Autodesk Inventor part; units mm, degrees
(part 7 of 13)
  line L2860 (13.767, 1.3537) -> (13.3324, 0.9191) construction
  line L2861 (13.3324, 0.9191) -> (13.3324, 0.3832) construction
  spline S914 degree 3 poles (13.3324, 0.3832) (13.3324, -0.1529) (13.767, -0.5874) (14.303, -0.5874) knots 0 0 0 0 1 1 1 1
  line L2862 (13.3324, 0.3832) -> (13.3324, -0.1529) construction
  line L2863 (13.3324, -0.1529) -> (13.767, -0.5874) construction
  line L2864 (13.767, -0.5874) -> (14.303, -0.5874) construction
  spline S915 degree 3 poles (14.303, -0.5874) (14.839, -0.5874) (15.2735, -0.1529) (15.2735, 0.3832) knots 0 0 0 0 1 1 1 1
  line L2865 (14.303, -0.5874) -> (14.839, -0.5874) construction
  line L2866 (14.839, -0.5874) -> (15.2735, -0.1529) construction
  line L2867 (15.2735, -0.1529) -> (15.2735, 0.3832) construction
  spline S916 degree 3 poles (17.8276, 0.3832) (17.8276, 0.9191) (17.3931, 1.3537) (16.8571, 1.3537) knots 0 0 0 0 1 1 1 1
  line L2868 (17.8276, 0.3832) -> (17.8276, 0.9191) construction
  line L2869 (17.8276, 0.9191) -> (17.3931, 1.3537) construction
  line L2870 (17.3931, 1.3537) -> (16.8571, 1.3537) construction
  spline S917 degree 3 poles (16.8571, 1.3537) (16.3211, 1.3537) (15.8866, 0.9191) (15.8866, 0.3832) knots 0 0 0 0 1 1 1 1
  line L2871 (16.8571, 1.3537) -> (16.3211, 1.3537) construction
  line L2872 (16.3211, 1.3537) -> (15.8866, 0.9191) construction
  line L2873 (15.8866, 0.9191) -> (15.8866, 0.3832) construction
  spline S918 degree 3 poles (15.8866, 0.3832) (15.8866, -0.1529) (16.3211, -0.5874) (16.8571, -0.5874) knots 0 0 0 0 1 1 1 1
  line L2874 (15.8866, 0.3832) -> (15.8866, -0.1529) construction
  line L2875 (15.8866, -0.1529) -> (16.3211, -0.5874) construction
  line L2876 (16.3211, -0.5874) -> (16.8571, -0.5874) construction
  spline S919 degree 3 poles (16.8571, -0.5874) (17.3931, -0.5874) (17.8276, -0.1529) (17.8276, 0.3832) knots 0 0 0 0 1 1 1 1
  line L2877 (16.8571, -0.5874) -> (17.3931, -0.5874) construction
  line L2878 (17.3931, -0.5874) -> (17.8276, -0.1529) construction
  line L2879 (17.8276, -0.1529) -> (17.8276, 0.3832) construction
  spline S920 degree 3 poles (17.8276, 2.9373) (17.8276, 3.4732) (17.3931, 3.9078) (16.8571, 3.9078) knots 0 0 0 0 1 1 1 1
  line L2880 (17.8276, 2.9373) -> (17.8276, 3.4732) construction
  line L2881 (17.8276, 3.4732) -> (17.3931, 3.9078) construction
  line L2882 (17.3931, 3.9078) -> (16.8571, 3.9078) construction
  spline S921 degree 3 poles (16.8571, 3.9078) (16.3211, 3.9078) (15.8866, 3.4732) (15.8866, 2.9373) knots 0 0 0 0 1 1 1 1
  line L2883 (16.8571, 3.9078) -> (16.3211, 3.9078) construction
  line L2884 (16.3211, 3.9078) -> (15.8866, 3.4732) construction
  line L2885 (15.8866, 3.4732) -> (15.8866, 2.9373) construction
  spline S922 degree 3 poles (15.8866, 2.9373) (15.8866, 2.4013) (16.3211, 1.9667) (16.8571, 1.9667) knots 0 0 0 0 1 1 1 1
  line L2886 (15.8866, 2.9373) -> (15.8866, 2.4013) construction
  line L2887 (15.8866, 2.4013) -> (16.3211, 1.9667) construction
  line L2888 (16.3211, 1.9667) -> (16.8571, 1.9667) construction
  spline S923 degree 3 poles (16.8571, 1.9667) (17.3931, 1.9667) (17.8276, 2.4013) (17.8276, 2.9373) knots 0 0 0 0 1 1 1 1
  line L2889 (16.8571, 1.9667) -> (17.3931, 1.9667) construction
  line L2890 (17.3931, 1.9667) -> (17.8276, 2.4013) construction
  line L2891 (17.8276, 2.4013) -> (17.8276, 2.9373) construction
  spline S924 degree 3 poles (20.3818, 2.9373) (20.3818, 3.4732) (19.9472, 3.9078) (19.4112, 3.9078) knots 0 0 0 0 1 1 1 1
  line L2892 (20.3818, 2.9373) -> (20.3818, 3.4732) construction
  line L2893 (20.3818, 3.4732) -> (19.9472, 3.9078) construction
  line L2894 (19.9472, 3.9078) -> (19.4112, 3.9078) construction
  spline S925 degree 3 poles (19.4112, 3.9078) (18.8752, 3.9078) (18.4407, 3.4732) (18.4407, 2.9373) knots 0 0 0 0 1 1 1 1
  line L2895 (19.4112, 3.9078) -> (18.8752, 3.9078) construction
  line L2896 (18.8752, 3.9078) -> (18.4407, 3.4732) construction
  line L2897 (18.4407, 3.4732) -> (18.4407, 2.9373) construction
  spline S926 degree 3 poles (18.4407, 2.9373) (18.4407, 2.4013) (18.8752, 1.9667) (19.4112, 1.9667) knots 0 0 0 0 1 1 1 1
  line L2898 (18.4407, 2.9373) -> (18.4407, 2.4013) construction
  line L2899 (18.4407, 2.4013) -> (18.8752, 1.9667) construction
  line L2900 (18.8752, 1.9667) -> (19.4112, 1.9667) construction
  spline S927 degree 3 poles (19.4112, 1.9667) (19.9472, 1.9667) (20.3818, 2.4013) (20.3818, 2.9373) knots 0 0 0 0 1 1 1 1
  line L2901 (19.4112, 1.9667) -> (19.9472, 1.9667) construction
  line L2902 (19.9472, 1.9667) -> (20.3818, 2.4013) construction
  line L2903 (20.3818, 2.4013) -> (20.3818, 2.9373) construction
  spline S928 degree 3 poles (26.767, 0.3832) (26.767, 0.9191) (26.3325, 1.3537) (25.7965, 1.3537) knots 0 0 0 0 1 1 1 1
  line L2904 (26.767, 0.3832) -> (26.767, 0.9191) construction
  line L2905 (26.767, 0.9191) -> (26.3325, 1.3537) construction
  line L2906 (26.3325, 1.3537) -> (25.7965, 1.3537) construction
  spline S929 degree 3 poles (25.7965, 1.3537) (25.2605, 1.3537) (24.8259, 0.9191) (24.8259, 0.3832) knots 0 0 0 0 1 1 1 1
  line L2907 (25.7965, 1.3537) -> (25.2605, 1.3537) construction
  line L2908 (25.2605, 1.3537) -> (24.8259, 0.9191) construction
  line L2909 (24.8259, 0.9191) -> (24.8259, 0.3832) construction
  spline S930 degree 3 poles (24.8259, 0.3832) (24.8259, -0.1529) (25.2605, -0.5874) (25.7965, -0.5874) knots 0 0 0 0 1 1 1 1
  line L2910 (24.8259, 0.3832) -> (24.8259, -0.1529) construction
  line L2911 (24.8259, -0.1529) -> (25.2605, -0.5874) construction
  line L2912 (25.2605, -0.5874) -> (25.7965, -0.5874) construction
  spline S931 degree 3 poles (25.7965, -0.5874) (26.3325, -0.5874) (26.767, -0.1529) (26.767, 0.3832) knots 0 0 0 0 1 1 1 1
  line L2913 (25.7965, -0.5874) -> (26.3325, -0.5874) construction
  line L2914 (26.3325, -0.5874) -> (26.767, -0.1529) construction
  line L2915 (26.767, -0.1529) -> (26.767, 0.3832) construction
  spline S932 degree 3 poles (24.2129, 0.3832) (24.2129, 0.9191) (23.7784, 1.3537) (23.2424, 1.3537) knots 0 0 0 0 1 1 1 1
  line L2916 (24.2129, 0.3832) -> (24.2129, 0.9191) construction
  line L2917 (24.2129, 0.9191) -> (23.7784, 1.3537) construction
  line L2918 (23.7784, 1.3537) -> (23.2424, 1.3537) construction
  spline S933 degree 3 poles (23.2424, 1.3537) (22.7064, 1.3537) (22.2718, 0.9191) (22.2718, 0.3832) knots 0 0 0 0 1 1 1 1
  line L2919 (23.2424, 1.3537) -> (22.7064, 1.3537) construction
  line L2920 (22.7064, 1.3537) -> (22.2718, 0.9191) construction
  line L2921 (22.2718, 0.9191) -> (22.2718, 0.3832) construction
  spline S934 degree 3 poles (22.2718, 0.3832) (22.2718, -0.1529) (22.7064, -0.5874) (23.2424, -0.5874) knots 0 0 0 0 1 1 1 1
  line L2922 (22.2718, 0.3832) -> (22.2718, -0.1529) construction
  line L2923 (22.2718, -0.1529) -> (22.7064, -0.5874) construction
  line L2924 (22.7064, -0.5874) -> (23.2424, -0.5874) construction
  spline S935 degree 3 poles (23.2424, -0.5874) (23.7784, -0.5874) (24.2129, -0.1529) (24.2129, 0.3832) knots 0 0 0 0 1 1 1 1
  line L2925 (23.2424, -0.5874) -> (23.7784, -0.5874) construction
  line L2926 (23.7784, -0.5874) -> (24.2129, -0.1529) construction
  line L2927 (24.2129, -0.1529) -> (24.2129, 0.3832) construction
  spline S936 degree 3 poles (21.6588, 0.3832) (21.6588, 0.9191) (21.2243, 1.3537) (20.6882, 1.3537) knots 0 0 0 0 1 1 1 1
  line L2928 (21.6588, 0.3832) -> (21.6588, 0.9191) construction
  line L2929 (21.6588, 0.9191) -> (21.2243, 1.3537) construction
  line L2930 (21.2243, 1.3537) -> (20.6882, 1.3537) construction
  spline S937 degree 3 poles (20.6882, 1.3537) (20.1523, 1.3537) (19.7177, 0.9191) (19.7177, 0.3832) knots 0 0 0 0 1 1 1 1
  line L2931 (20.6882, 1.3537) -> (20.1523, 1.3537) construction
  line L2932 (20.1523, 1.3537) -> (19.7177, 0.9191) construction
  line L2933 (19.7177, 0.9191) -> (19.7177, 0.3832) construction
  spline S938 degree 3 poles (19.7177, 0.3832) (19.7177, -0.1529) (20.1523, -0.5874) (20.6882, -0.5874) knots 0 0 0 0 1 1 1 1
  line L2934 (19.7177, 0.3832) -> (19.7177, -0.1529) construction
  line L2935 (19.7177, -0.1529) -> (20.1523, -0.5874) construction
  line L2936 (20.1523, -0.5874) -> (20.6882, -0.5874) construction
  spline S939 degree 3 poles (20.6882, -0.5874) (21.2243, -0.5874) (21.6588, -0.1529) (21.6588, 0.3832) knots 0 0 0 0 1 1 1 1
  line L2937 (20.6882, -0.5874) -> (21.2243, -0.5874) construction
  line L2938 (21.2243, -0.5874) -> (21.6588, -0.1529) construction
  line L2939 (21.6588, -0.1529) -> (21.6588, 0.3832) construction
  spline S940 degree 3 poles (20.3818, 5.4914) (20.3818, 6.0273) (19.9472, 6.4619) (19.4112, 6.4619) knots 0 0 0 0 1 1 1 1
  line L2940 (20.3818, 5.4914) -> (20.3818, 6.0273) construction
  line L2941 (20.3818, 6.0273) -> (19.9472, 6.4619) construction
  line L2942 (19.9472, 6.4619) -> (19.4112, 6.4619) construction
  spline S941 degree 3 poles (19.4112, 6.4619) (18.8752, 6.4619) (18.4407, 6.0273) (18.4407, 5.4914) knots 0 0 0 0 1 1 1 1
  line L2943 (19.4112, 6.4619) -> (18.8752, 6.4619) construction
  line L2944 (18.8752, 6.4619) -> (18.4407, 6.0273) construction
  line L2945 (18.4407, 6.0273) -> (18.4407, 5.4914) construction
  spline S942 degree 3 poles (18.4407, 5.4914) (18.4407, 4.9554) (18.8752, 4.5208) (19.4112, 4.5208) knots 0 0 0 0 1 1 1 1
  line L2946 (18.4407, 5.4914) -> (18.4407, 4.9554) construction
  line L2947 (18.4407, 4.9554) -> (18.8752, 4.5208) construction
  line L2948 (18.8752, 4.5208) -> (19.4112, 4.5208) construction
  spline S943 degree 3 poles (19.4112, 4.5208) (19.9472, 4.5208) (20.3818, 4.9554) (20.3818, 5.4914) knots 0 0 0 0 1 1 1 1
  line L2949 (19.4112, 4.5208) -> (19.9472, 4.5208) construction
  line L2950 (19.9472, 4.5208) -> (20.3818, 4.9554) construction
  line L2951 (20.3818, 4.9554) -> (20.3818, 5.4914) construction
  spline S944 degree 3 poles (20.3818, 8.0455) (20.3818, 8.5815) (19.9472, 9.016) (19.4112, 9.016) knots 0 0 0 0 1 1 1 1
  line L2952 (20.3818, 8.0455) -> (20.3818, 8.5815) construction
  line L2953 (20.3818, 8.5815) -> (19.9472, 9.016) construction
  line L2954 (19.9472, 9.016) -> (19.4112, 9.016) construction
  spline S945 degree 3 poles (19.4112, 9.016) (18.8752, 9.016) (18.4407, 8.5815) (18.4407, 8.0455) knots 0 0 0 0 1 1 1 1
  line L2955 (19.4112, 9.016) -> (18.8752, 9.016) construction
  line L2956 (18.8752, 9.016) -> (18.4407, 8.5815) construction
  line L2957 (18.4407, 8.5815) -> (18.4407, 8.0455) construction
  spline S946 degree 3 poles (18.4407, 8.0455) (18.4407, 7.5095) (18.8752, 7.0749) (19.4112, 7.0749) knots 0 0 0 0 1 1 1 1
  line L2958 (18.4407, 8.0455) -> (18.4407, 7.5095) construction
  line L2959 (18.4407, 7.5095) -> (18.8752, 7.0749) construction
  line L2960 (18.8752, 7.0749) -> (19.4112, 7.0749) construction
  spline S947 degree 3 poles (19.4112, 7.0749) (19.9472, 7.0749) (20.3818, 7.5095) (20.3818, 8.0455) knots 0 0 0 0 1 1 1 1
  line L2961 (19.4112, 7.0749) -> (19.9472, 7.0749) construction
  line L2962 (19.9472, 7.0749) -> (20.3818, 7.5095) construction
  line L2963 (20.3818, 7.5095) -> (20.3818, 8.0455) construction
  spline S948 degree 3 poles (20.3818, 10.5996) (20.3818, 11.1356) (19.9472, 11.5701) (19.4112, 11.5701) knots 0 0 0 0 1 1 1 1
  line L2964 (20.3818, 10.5996) -> (20.3818, 11.1356) construction
  line L2965 (20.3818, 11.1356) -> (19.9472, 11.5701) construction
  line L2966 (19.9472, 11.5701) -> (19.4112, 11.5701) construction
  spline S949 degree 3 poles (19.4112, 11.5701) (18.8752, 11.5701) (18.4407, 11.1356) (18.4407, 10.5996) knots 0 0 0 0 1 1 1 1
  line L2967 (19.4112, 11.5701) -> (18.8752, 11.5701) construction
  line L2968 (18.8752, 11.5701) -> (18.4407, 11.1356) construction
  line L2969 (18.4407, 11.1356) -> (18.4407, 10.5996) construction
  spline S950 degree 3 poles (18.4407, 10.5996) (18.4407, 10.0636) (18.8752, 9.629) (19.4112, 9.629) knots 0 0 0 0 1 1 1 1
  line L2970 (18.4407, 10.5996) -> (18.4407, 10.0636) construction
  line L2971 (18.4407, 10.0636) -> (18.8752, 9.629) construction
  line L2972 (18.8752, 9.629) -> (19.4112, 9.629) construction
  spline S951 degree 3 poles (19.4112, 9.629) (19.9472, 9.629) (20.3818, 10.0636) (20.3818, 10.5996) knots 0 0 0 0 1 1 1 1
  line L2973 (19.4112, 9.629) -> (19.9472, 9.629) construction
  line L2974 (19.9472, 9.629) -> (20.3818, 10.0636) construction
  line L2975 (20.3818, 10.0636) -> (20.3818, 10.5996) construction
  spline S952 degree 3 poles (23.319, 11.7489) (23.319, 12.2849) (22.8844, 12.7194) (22.3485, 12.7194) knots 0 0 0 0 1 1 1 1
  line L2976 (23.319, 11.7489) -> (23.319, 12.2849) construction
  line L2977 (23.319, 12.2849) -> (22.8844, 12.7194) construction
  line L2978 (22.8844, 12.7194) -> (22.3485, 12.7194) construction
  spline S953 degree 3 poles (22.3485, 12.7194) (21.8125, 12.7194) (21.3779, 12.2849) (21.3779, 11.7489) knots 0 0 0 0 1 1 1 1
  line L2979 (22.3485, 12.7194) -> (21.8125, 12.7194) construction
  line L2980 (21.8125, 12.7194) -> (21.3779, 12.2849) construction
  line L2981 (21.3779, 12.2849) -> (21.3779, 11.7489) construction
  spline S954 degree 3 poles (21.3779, 11.7489) (21.3779, 11.2129) (21.8125, 10.7783) (22.3485, 10.7783) knots 0 0 0 0 1 1 1 1
  line L2982 (21.3779, 11.7489) -> (21.3779, 11.2129) construction
  line L2983 (21.3779, 11.2129) -> (21.8125, 10.7783) construction
  line L2984 (21.8125, 10.7783) -> (22.3485, 10.7783) construction
  spline S955 degree 3 poles (22.3485, 10.7783) (22.8844, 10.7783) (23.319, 11.2129) (23.319, 11.7489) knots 0 0 0 0 1 1 1 1
  line L2985 (22.3485, 10.7783) -> (22.8844, 10.7783) construction
  line L2986 (22.8844, 10.7783) -> (23.319, 11.2129) construction
  line L2987 (23.319, 11.2129) -> (23.319, 11.7489) construction
  spline S956 degree 3 poles (25.8731, 11.7489) (25.8731, 12.2849) (25.4385, 12.7194) (24.9026, 12.7194) knots 0 0 0 0 1 1 1 1
  line L2988 (25.8731, 11.7489) -> (25.8731, 12.2849) construction
  line L2989 (25.8731, 12.2849) -> (25.4385, 12.7194) construction
  line L2990 (25.4385, 12.7194) -> (24.9026, 12.7194) construction
  spline S957 degree 3 poles (24.9026, 12.7194) (24.3666, 12.7194) (23.932, 12.2849) (23.932, 11.7489) knots 0 0 0 0 1 1 1 1
  line L2991 (24.9026, 12.7194) -> (24.3666, 12.7194) construction
  line L2992 (24.3666, 12.7194) -> (23.932, 12.2849) construction
  line L2993 (23.932, 12.2849) -> (23.932, 11.7489) construction
  spline S958 degree 3 poles (23.932, 11.7489) (23.932, 11.2129) (24.3666, 10.7783) (24.9026, 10.7783) knots 0 0 0 0 1 1 1 1
  line L2994 (23.932, 11.7489) -> (23.932, 11.2129) construction
  line L2995 (23.932, 11.2129) -> (24.3666, 10.7783) construction
  line L2996 (24.3666, 10.7783) -> (24.9026, 10.7783) construction
  spline S959 degree 3 poles (24.9026, 10.7783) (25.4385, 10.7783) (25.8731, 11.2129) (25.8731, 11.7489) knots 0 0 0 0 1 1 1 1
  line L2997 (24.9026, 10.7783) -> (25.4385, 10.7783) construction
  line L2998 (25.4385, 10.7783) -> (25.8731, 11.2129) construction
  line L2999 (25.8731, 11.2129) -> (25.8731, 11.7489) construction
  spline S960 degree 3 poles (23.319, 14.303) (23.319, 14.839) (22.8844, 15.2735) (22.3485, 15.2735) knots 0 0 0 0 1 1 1 1
  line L3000 (23.319, 14.303) -> (23.319, 14.839) construction
  line L3001 (23.319, 14.839) -> (22.8844, 15.2735) construction
  line L3002 (22.8844, 15.2735) -> (22.3485, 15.2735) construction
  spline S961 degree 3 poles (22.3485, 15.2735) (21.8125, 15.2735) (21.3779, 14.839) (21.3779, 14.303) knots 0 0 0 0 1 1 1 1
  line L3003 (22.3485, 15.2735) -> (21.8125, 15.2735) construction
  line L3004 (21.8125, 15.2735) -> (21.3779, 14.839) construction
  line L3005 (21.3779, 14.839) -> (21.3779, 14.303) construction
  spline S962 degree 3 poles (21.3779, 14.303) (21.3779, 13.767) (21.8125, 13.3324) (22.3485, 13.3324) knots 0 0 0 0 1 1 1 1
  line L3006 (21.3779, 14.303) -> (21.3779, 13.767) construction
  line L3007 (21.3779, 13.767) -> (21.8125, 13.3324) construction
  line L3008 (21.8125, 13.3324) -> (22.3485, 13.3324) construction
  spline S963 degree 3 poles (22.3485, 13.3324) (22.8844, 13.3324) (23.319, 13.767) (23.319, 14.303) knots 0 0 0 0 1 1 1 1
  line L3009 (22.3485, 13.3324) -> (22.8844, 13.3324) construction
  line L3010 (22.8844, 13.3324) -> (23.319, 13.767) construction
  line L3011 (23.319, 13.767) -> (23.319, 14.303) construction
  spline S964 degree 3 poles (25.8731, 14.303) (25.8731, 14.839) (25.4385, 15.2735) (24.9026, 15.2735) knots 0 0 0 0 1 1 1 1
  line L3012 (25.8731, 14.303) -> (25.8731, 14.839) construction
  line L3013 (25.8731, 14.839) -> (25.4385, 15.2735) construction
  line L3014 (25.4385, 15.2735) -> (24.9026, 15.2735) construction
  spline S965 degree 3 poles (24.9026, 15.2735) (24.3666, 15.2735) (23.932, 14.839) (23.932, 14.303) knots 0 0 0 0 1 1 1 1
  line L3015 (24.9026, 15.2735) -> (24.3666, 15.2735) construction
  line L3016 (24.3666, 15.2735) -> (23.932, 14.839) construction
  line L3017 (23.932, 14.839) -> (23.932, 14.303) construction
  spline S966 degree 3 poles (23.932, 14.303) (23.932, 13.767) (24.3666, 13.3324) (24.9026, 13.3324) knots 0 0 0 0 1 1 1 1
  line L3018 (23.932, 14.303) -> (23.932, 13.767) construction
  line L3019 (23.932, 13.767) -> (24.3666, 13.3324) construction
  line L3020 (24.3666, 13.3324) -> (24.9026, 13.3324) construction
  spline S967 degree 3 poles (24.9026, 13.3324) (25.4385, 13.3324) (25.8731, 13.767) (25.8731, 14.303) knots 0 0 0 0 1 1 1 1
  line L3021 (24.9026, 13.3324) -> (25.4385, 13.3324) construction
  line L3022 (25.4385, 13.3324) -> (25.8731, 13.767) construction
  line L3023 (25.8731, 13.767) -> (25.8731, 14.303) construction
  spline S968 degree 3 poles (17.8276, 5.4914) (17.8276, 6.0273) (17.3931, 6.4619) (16.8571, 6.4619) knots 0 0 0 0 1 1 1 1
  line L3024 (17.8276, 5.4914) -> (17.8276, 6.0273) construction
  line L3025 (17.8276, 6.0273) -> (17.3931, 6.4619) construction
  line L3026 (17.3931, 6.4619) -> (16.8571, 6.4619) construction
  spline S969 degree 3 poles (16.8571, 6.4619) (16.3211, 6.4619) (15.8866, 6.0273) (15.8866, 5.4914) knots 0 0 0 0 1 1 1 1
  line L3027 (16.8571, 6.4619) -> (16.3211, 6.4619) construction
  line L3028 (16.3211, 6.4619) -> (15.8866, 6.0273) construction
  line L3029 (15.8866, 6.0273) -> (15.8866, 5.4914) construction
  spline S970 degree 3 poles (15.8866, 5.4914) (15.8866, 4.9554) (16.3211, 4.5208) (16.8571, 4.5208) knots 0 0 0 0 1 1 1 1
  line L3030 (15.8866, 5.4914) -> (15.8866, 4.9554) construction
  line L3031 (15.8866, 4.9554) -> (16.3211, 4.5208) construction
  line L3032 (16.3211, 4.5208) -> (16.8571, 4.5208) construction
  spline S971 degree 3 poles (16.8571, 4.5208) (17.3931, 4.5208) (17.8276, 4.9554) (17.8276, 5.4914) knots 0 0 0 0 1 1 1 1
  line L3033 (16.8571, 4.5208) -> (17.3931, 4.5208) construction
  line L3034 (17.3931, 4.5208) -> (17.8276, 4.9554) construction
  line L3035 (17.8276, 4.9554) -> (17.8276, 5.4914) construction
  spline S972 degree 3 poles (17.8276, 8.0455) (17.8276, 8.5815) (17.3931, 9.016) (16.8571, 9.016) knots 0 0 0 0 1 1 1 1
  line L3036 (17.8276, 8.0455) -> (17.8276, 8.5815) construction
  line L3037 (17.8276, 8.5815) -> (17.3931, 9.016) construction
  line L3038 (17.3931, 9.016) -> (16.8571, 9.016) construction
  spline S973 degree 3 poles (16.8571, 9.016) (16.3211, 9.016) (15.8866, 8.5815) (15.8866, 8.0455) knots 0 0 0 0 1 1 1 1
  line L3039 (16.8571, 9.016) -> (16.3211, 9.016) construction
  line L3040 (16.3211, 9.016) -> (15.8866, 8.5815) construction
  line L3041 (15.8866, 8.5815) -> (15.8866, 8.0455) construction
  spline S974 degree 3 poles (15.8866, 8.0455) (15.8866, 7.5095) (16.3211, 7.0749) (16.8571, 7.0749) knots 0 0 0 0 1 1 1 1
  line L3042 (15.8866, 8.0455) -> (15.8866, 7.5095) construction
  line L3043 (15.8866, 7.5095) -> (16.3211, 7.0749) construction
  line L3044 (16.3211, 7.0749) -> (16.8571, 7.0749) construction
  spline S975 degree 3 poles (16.8571, 7.0749) (17.3931, 7.0749) (17.8276, 7.5095) (17.8276, 8.0455) knots 0 0 0 0 1 1 1 1
  line L3045 (16.8571, 7.0749) -> (17.3931, 7.0749) construction
  line L3046 (17.3931, 7.0749) -> (17.8276, 7.5095) construction
  line L3047 (17.8276, 7.5095) -> (17.8276, 8.0455) construction
  spline S976 degree 3 poles (17.8276, 10.5996) (17.8276, 11.1356) (17.3931, 11.5701) (16.8571, 11.5701) knots 0 0 0 0 1 1 1 1
  line L3048 (17.8276, 10.5996) -> (17.8276, 11.1356) construction
  line L3049 (17.8276, 11.1356) -> (17.3931, 11.5701) construction
  line L3050 (17.3931, 11.5701) -> (16.8571, 11.5701) construction
  spline S977 degree 3 poles (16.8571, 11.5701) (16.3211, 11.5701) (15.8866, 11.1356) (15.8866, 10.5996) knots 0 0 0 0 1 1 1 1
  line L3051 (16.8571, 11.5701) -> (16.3211, 11.5701) construction
  line L3052 (16.3211, 11.5701) -> (15.8866, 11.1356) construction
  line L3053 (15.8866, 11.1356) -> (15.8866, 10.5996) construction
  spline S978 degree 3 poles (15.8866, 10.5996) (15.8866, 10.0636) (16.3211, 9.629) (16.8571, 9.629) knots 0 0 0 0 1 1 1 1
  line L3054 (15.8866, 10.5996) -> (15.8866, 10.0636) construction
  line L3055 (15.8866, 10.0636) -> (16.3211, 9.629) construction
  line L3056 (16.3211, 9.629) -> (16.8571, 9.629) construction
  spline S979 degree 3 poles (16.8571, 9.629) (17.3931, 9.629) (17.8276, 10.0636) (17.8276, 10.5996) knots 0 0 0 0 1 1 1 1
  line L3057 (16.8571, 9.629) -> (17.3931, 9.629) construction
  line L3058 (17.3931, 9.629) -> (17.8276, 10.0636) construction
  line L3059 (17.8276, 10.0636) -> (17.8276, 10.5996) construction
  spline S980 degree 3 poles (17.8276, 13.1537) (17.8276, 13.6897) (17.3931, 14.1242) (16.8571, 14.1242) knots 0 0 0 0 1 1 1 1
  line L3060 (17.8276, 13.1537) -> (17.8276, 13.6897) construction
  line L3061 (17.8276, 13.6897) -> (17.3931, 14.1242) construction
  line L3062 (17.3931, 14.1242) -> (16.8571, 14.1242) construction
  spline S981 degree 3 poles (16.8571, 14.1242) (16.3211, 14.1242) (15.8866, 13.6897) (15.8866, 13.1537) knots 0 0 0 0 1 1 1 1
  line L3063 (16.8571, 14.1242) -> (16.3211, 14.1242) construction
  line L3064 (16.3211, 14.1242) -> (15.8866, 13.6897) construction
  line L3065 (15.8866, 13.6897) -> (15.8866, 13.1537) construction
  spline S982 degree 3 poles (15.8866, 13.1537) (15.8866, 12.6177) (16.3211, 12.1831) (16.8571, 12.1831) knots 0 0 0 0 1 1 1 1
  line L3066 (15.8866, 13.1537) -> (15.8866, 12.6177) construction
  line L3067 (15.8866, 12.6177) -> (16.3211, 12.1831) construction
  line L3068 (16.3211, 12.1831) -> (16.8571, 12.1831) construction
  spline S983 degree 3 poles (16.8571, 12.1831) (17.3931, 12.1831) (17.8276, 12.6177) (17.8276, 13.1537) knots 0 0 0 0 1 1 1 1
  line L3069 (16.8571, 12.1831) -> (17.3931, 12.1831) construction
  line L3070 (17.3931, 12.1831) -> (17.8276, 12.6177) construction
  line L3071 (17.8276, 12.6177) -> (17.8276, 13.1537) construction
  spline S984 degree 3 poles (17.8276, 15.7078) (17.8276, 16.2438) (17.3931, 16.6783) (16.8571, 16.6783) knots 0 0 0 0 1 1 1 1
  line L3072 (17.8276, 15.7078) -> (17.8276, 16.2438) construction
  line L3073 (17.8276, 16.2438) -> (17.3931, 16.6783) construction
  line L3074 (17.3931, 16.6783) -> (16.8571, 16.6783) construction
  spline S985 degree 3 poles (16.8571, 16.6783) (16.3211, 16.6783) (15.8866, 16.2438) (15.8866, 15.7078) knots 0 0 0 0 1 1 1 1
  line L3075 (16.8571, 16.6783) -> (16.3211, 16.6783) construction
  line L3076 (16.3211, 16.6783) -> (15.8866, 16.2438) construction
  line L3077 (15.8866, 16.2438) -> (15.8866, 15.7078) construction
  spline S986 degree 3 poles (15.8866, 15.7078) (15.8866, 15.1718) (16.3211, 14.7372) (16.8571, 14.7372) knots 0 0 0 0 1 1 1 1
  line L3078 (15.8866, 15.7078) -> (15.8866, 15.1718) construction
  line L3079 (15.8866, 15.1718) -> (16.3211, 14.7372) construction
  line L3080 (16.3211, 14.7372) -> (16.8571, 14.7372) construction
  spline S987 degree 3 poles (16.8571, 14.7372) (17.3931, 14.7372) (17.8276, 15.1718) (17.8276, 15.7078) knots 0 0 0 0 1 1 1 1
  line L3081 (16.8571, 14.7372) -> (17.3931, 14.7372) construction
  line L3082 (17.3931, 14.7372) -> (17.8276, 15.1718) construction
  line L3083 (17.8276, 15.1718) -> (17.8276, 15.7078) construction
  spline S988 degree 3 poles (17.8276, 18.2619) (17.8276, 18.7979) (17.3931, 19.2324) (16.8571, 19.2324) knots 0 0 0 0 1 1 1 1
  line L3084 (17.8276, 18.2619) -> (17.8276, 18.7979) construction
  line L3085 (17.8276, 18.7979) -> (17.3931, 19.2324) construction
  line L3086 (17.3931, 19.2324) -> (16.8571, 19.2324) construction
  spline S989 degree 3 poles (16.8571, 19.2324) (16.3211, 19.2324) (15.8866, 18.7979) (15.8866, 18.2619) knots 0 0 0 0 1 1 1 1
  line L3087 (16.8571, 19.2324) -> (16.3211, 19.2324) construction
  line L3088 (16.3211, 19.2324) -> (15.8866, 18.7979) construction
  line L3089 (15.8866, 18.7979) -> (15.8866, 18.2619) construction
  spline S990 degree 3 poles (15.8866, 18.2619) (15.8866, 17.7259) (16.3211, 17.2914) (16.8571, 17.2914) knots 0 0 0 0 1 1 1 1
  line L3090 (15.8866, 18.2619) -> (15.8866, 17.7259) construction
  line L3091 (15.8866, 17.7259) -> (16.3211, 17.2914) construction
  line L3092 (16.3211, 17.2914) -> (16.8571, 17.2914) construction
  spline S991 degree 3 poles (16.8571, 17.2914) (17.3931, 17.2914) (17.8276, 17.7259) (17.8276, 18.2619) knots 0 0 0 0 1 1 1 1
  line L3093 (16.8571, 17.2914) -> (17.3931, 17.2914) construction
  line L3094 (17.3931, 17.2914) -> (17.8276, 17.7259) construction
  line L3095 (17.8276, 17.7259) -> (17.8276, 18.2619) construction
  spline S992 degree 3 poles (17.8276, 20.816) (17.8276, 21.352) (17.3931, 21.7866) (16.8571, 21.7866) knots 0 0 0 0 1 1 1 1
  line L3096 (17.8276, 20.816) -> (17.8276, 21.352) construction
  line L3097 (17.8276, 21.352) -> (17.3931, 21.7866) construction
  line L3098 (17.3931, 21.7866) -> (16.8571, 21.7866) construction
  spline S993 degree 3 poles (16.8571, 21.7866) (16.3211, 21.7866) (15.8866, 21.352) (15.8866, 20.816) knots 0 0 0 0 1 1 1 1
  line L3099 (16.8571, 21.7866) -> (16.3211, 21.7866) construction
  line L3100 (16.3211, 21.7866) -> (15.8866, 21.352) construction
  line L3101 (15.8866, 21.352) -> (15.8866, 20.816) construction
  spline S994 degree 3 poles (15.8866, 20.816) (15.8866, 20.28) (16.3211, 19.8455) (16.8571, 19.8455) knots 0 0 0 0 1 1 1 1
  line L3102 (15.8866, 20.816) -> (15.8866, 20.28) construction
  line L3103 (15.8866, 20.28) -> (16.3211, 19.8455) construction
  line L3104 (16.3211, 19.8455) -> (16.8571, 19.8455) construction
  spline S995 degree 3 poles (16.8571, 19.8455) (17.3931, 19.8455) (17.8276, 20.28) (17.8276, 20.816) knots 0 0 0 0 1 1 1 1
  line L3105 (16.8571, 19.8455) -> (17.3931, 19.8455) construction
  line L3106 (17.3931, 19.8455) -> (17.8276, 20.28) construction
  line L3107 (17.8276, 20.28) -> (17.8276, 20.816) construction
  spline S996 degree 3 poles (20.3818, 13.1537) (20.3818, 13.6897) (19.9472, 14.1242) (19.4112, 14.1242) knots 0 0 0 0 1 1 1 1
  line L3108 (20.3818, 13.1537) -> (20.3818, 13.6897) construction
  line L3109 (20.3818, 13.6897) -> (19.9472, 14.1242) construction
  line L3110 (19.9472, 14.1242) -> (19.4112, 14.1242) construction
  spline S997 degree 3 poles (19.4112, 14.1242) (18.8752, 14.1242) (18.4407, 13.6897) (18.4407, 13.1537) knots 0 0 0 0 1 1 1 1
  line L3111 (19.4112, 14.1242) -> (18.8752, 14.1242) construction
  line L3112 (18.8752, 14.1242) -> (18.4407, 13.6897) construction
  line L3113 (18.4407, 13.6897) -> (18.4407, 13.1537) construction
  spline S998 degree 3 poles (18.4407, 13.1537) (18.4407, 12.6177) (18.8752, 12.1831) (19.4112, 12.1831) knots 0 0 0 0 1 1 1 1
  line L3114 (18.4407, 13.1537) -> (18.4407, 12.6177) construction
  line L3115 (18.4407, 12.6177) -> (18.8752, 12.1831) construction
  line L3116 (18.8752, 12.1831) -> (19.4112, 12.1831) construction
  spline S999 degree 3 poles (19.4112, 12.1831) (19.9472, 12.1831) (20.3818, 12.6177) (20.3818, 13.1537) knots 0 0 0 0 1 1 1 1
  line L3117 (19.4112, 12.1831) -> (19.9472, 12.1831) construction
  line L3118 (19.9472, 12.1831) -> (20.3818, 12.6177) construction
  line L3119 (20.3818, 12.6177) -> (20.3818, 13.1537) construction
  spline S1000 degree 3 poles (20.3818, 15.7078) (20.3818, 16.2438) (19.9472, 16.6783) (19.4112, 16.6783) knots 0 0 0 0 1 1 1 1
  line L3120 (20.3818, 15.7078) -> (20.3818, 16.2438) construction
  line L3121 (20.3818, 16.2438) -> (19.9472, 16.6783) construction
  line L3122 (19.9472, 16.6783) -> (19.4112, 16.6783) construction
  spline S1001 degree 3 poles (19.4112, 16.6783) (18.8752, 16.6783) (18.4407, 16.2438) (18.4407, 15.7078) knots 0 0 0 0 1 1 1 1
  line L3123 (19.4112, 16.6783) -> (18.8752, 16.6783) construction
  line L3124 (18.8752, 16.6783) -> (18.4407, 16.2438) construction
  line L3125 (18.4407, 16.2438) -> (18.4407, 15.7078) construction
  spline S1002 degree 3 poles (18.4407, 15.7078) (18.4407, 15.1718) (18.8752, 14.7372) (19.4112, 14.7372) knots 0 0 0 0 1 1 1 1
  line L3126 (18.4407, 15.7078) -> (18.4407, 15.1718) construction
  line L3127 (18.4407, 15.1718) -> (18.8752, 14.7372) construction
  line L3128 (18.8752, 14.7372) -> (19.4112, 14.7372) construction
  spline S1003 degree 3 poles (19.4112, 14.7372) (19.9472, 14.7372) (20.3818, 15.1718) (20.3818, 15.7078) knots 0 0 0 0 1 1 1 1
  line L3129 (19.4112, 14.7372) -> (19.9472, 14.7372) construction
  line L3130 (19.9472, 14.7372) -> (20.3818, 15.1718) construction
  line L3131 (20.3818, 15.1718) -> (20.3818, 15.7078) construction
  spline S1004 degree 3 poles (20.3818, 18.2619) (20.3818, 18.7979) (19.9472, 19.2324) (19.4112, 19.2324) knots 0 0 0 0 1 1 1 1
  line L3132 (20.3818, 18.2619) -> (20.3818, 18.7979) construction
  line L3133 (20.3818, 18.7979) -> (19.9472, 19.2324) construction
  line L3134 (19.9472, 19.2324) -> (19.4112, 19.2324) construction
  spline S1005 degree 3 poles (19.4112, 19.2324) (18.8752, 19.2324) (18.4407, 18.7979) (18.4407, 18.2619) knots 0 0 0 0 1 1 1 1
  line L3135 (19.4112, 19.2324) -> (18.8752, 19.2324) construction
  line L3136 (18.8752, 19.2324) -> (18.4407, 18.7979) construction
  line L3137 (18.4407, 18.7979) -> (18.4407, 18.2619) construction
  spline S1006 degree 3 poles (18.4407, 18.2619) (18.4407, 17.7259) (18.8752, 17.2914) (19.4112, 17.2914) knots 0 0 0 0 1 1 1 1
  line L3138 (18.4407, 18.2619) -> (18.4407, 17.7259) construction
  line L3139 (18.4407, 17.7259) -> (18.8752, 17.2914) construction
  line L3140 (18.8752, 17.2914) -> (19.4112, 17.2914) construction
  spline S1007 degree 3 poles (19.4112, 17.2914) (19.9472, 17.2914) (20.3818, 17.7259) (20.3818, 18.2619) knots 0 0 0 0 1 1 1 1
  line L3141 (19.4112, 17.2914) -> (19.9472, 17.2914) construction
  line L3142 (19.9472, 17.2914) -> (20.3818, 17.7259) construction
  line L3143 (20.3818, 17.7259) -> (20.3818, 18.2619) construction
  spline S1008 degree 3 poles (20.3818, 20.816) (20.3818, 21.352) (19.9472, 21.7866) (19.4112, 21.7866) knots 0 0 0 0 1 1 1 1
  line L3144 (20.3818, 20.816) -> (20.3818, 21.352) construction
  line L3145 (20.3818, 21.352) -> (19.9472, 21.7866) construction
  line L3146 (19.9472, 21.7866) -> (19.4112, 21.7866) construction
  spline S1009 degree 3 poles (19.4112, 21.7866) (18.8752, 21.7866) (18.4407, 21.352) (18.4407, 20.816) knots 0 0 0 0 1 1 1 1
  line L3147 (19.4112, 21.7866) -> (18.8752, 21.7866) construction
  line L3148 (18.8752, 21.7866) -> (18.4407, 21.352) construction
  line L3149 (18.4407, 21.352) -> (18.4407, 20.816) construction
  spline S1010 degree 3 poles (18.4407, 20.816) (18.4407, 20.28) (18.8752, 19.8455) (19.4112, 19.8455) knots 0 0 0 0 1 1 1 1
  line L3150 (18.4407, 20.816) -> (18.4407, 20.28) construction
  line L3151 (18.4407, 20.28) -> (18.8752, 19.8455) construction
  line L3152 (18.8752, 19.8455) -> (19.4112, 19.8455) construction
  spline S1011 degree 3 poles (19.4112, 19.8455) (19.9472, 19.8455) (20.3818, 20.28) (20.3818, 20.816) knots 0 0 0 0 1 1 1 1
  line L3153 (19.4112, 19.8455) -> (19.9472, 19.8455) construction
  line L3154 (19.9472, 19.8455) -> (20.3818, 20.28) construction
  line L3155 (20.3818, 20.28) -> (20.3818, 20.816) construction
  line L3156 (20.0497, 10.5996) -> (19.4112, 10.5996)
  line L3157 (41.1212, 33.7142) -> (41.1212, 33.4588)
  line L3158 (38.567, 33.7142) -> (38.567, 33.4588)
  line L3159 (46.2294, 33.7142) -> (46.2294, 33.4588)
  line L3160 (47.5064, 34.4805) -> (37.29, 34.4805)
  line L3161 (47.5064, 32.6927) -> (37.29, 32.6927)
  line L3162 (43.6753, 33.7142) -> (43.6753, 33.4588)
  line L3163 (37.29, 16.6017) -> (34.7358, 16.6017)
  line L3164 (36.0129, 15.8354) -> (36.0129, 15.58)
  line L3165 (37.29, 17.368) -> (34.7358, 17.368)
  line L3166 (36.0129, 18.3895) -> (36.0129, 18.1341)
  line L3167 (37.29, 19.1558) -> (34.7358, 19.1558)
  line L3168 (37.29, 19.9221) -> (34.7358, 19.9221)
  line L3169 (37.29, 21.7099) -> (34.7358, 21.7099)
  line L3170 (36.0129, 20.9436) -> (36.0129, 20.6882)
  line L3171 (37.29, 22.4762) -> (34.7358, 22.4762)
  line L3172 (36.0129, 23.4977) -> (36.0129, 23.2424)
  line L3173 (37.29, 24.264) -> (34.7358, 24.264)
  line L3174 (37.29, 25.0303) -> (34.7358, 25.0303)
  line L3175 (37.29, 26.8181) -> (34.7358, 26.8181)
  line L3176 (36.0129, 26.0518) -> (36.0129, 25.7965)
  line L3177 (37.29, 27.5844) -> (34.7358, 27.5844)
  line L3178 (36.0129, 28.606) -> (36.0129, 28.3506)
  line L3179 (37.29, 29.3723) -> (34.7358, 29.3723)
  line L3180 (37.29, 30.1386) -> (34.7358, 30.1386)
  line L3181 (36.0129, 31.1601) -> (36.0129, 30.9047)
  line L3182 (16.8571, 32.6927) -> (6.6406, 32.6927)
  line L3183 (13.0259, 33.7142) -> (13.0259, 33.4588)
  line L3184 (10.4718, 33.7142) -> (10.4718, 33.4588)
  line L3185 (16.8571, 34.4805) -> (6.6406, 34.4805)
  line L3186 (15.58, 33.7142) -> (15.58, 33.4588)
  line L3187 (7.9177, 33.7142) -> (7.9177, 33.4588)
  line L3188 (18.1341, 31.1601) -> (18.1341, 30.9047)
  line L3189 (16.8571, -0.5108) -> (6.6406, -0.5108)
  line L3190 (13.0259, 0.5108) -> (13.0259, 0.2554)
  line L3191 (10.4718, 0.5108) -> (10.4718, 0.2554)
  line L3192 (16.8571, 1.2771) -> (6.6406, 1.2771)
  line L3193 (15.58, 0.5108) -> (15.58, 0.2554)
  line L3194 (7.9177, 0.5108) -> (7.9177, 0.2554)
  line L3195 (19.4112, 2.0434) -> (16.8571, 2.0434)
  line L3196 (18.1341, 3.0649) -> (18.1341, 2.8095)
  line L3197 (19.4112, 3.8312) -> (16.8571, 3.8312)
  line L3198 (19.4112, 4.5975) -> (16.8571, 4.5975)
  line L3199 (19.4112, 6.3853) -> (16.8571, 6.3853)
  line L3200 (18.1341, 5.619) -> (18.1341, 5.3636)
  line L3201 (19.4112, 7.1516) -> (16.8571, 7.1516)
  line L3202 (19.4112, 8.9394) -> (16.8571, 8.9394)
  line L3203 (19.4112, 9.7057) -> (16.8571, 9.7057)
  line L3204 (18.1341, 8.1731) -> (18.1341, 7.9177)
  line L3205 (19.4112, 11.4935) -> (16.8571, 11.4935)
  line L3206 (18.1341, 10.7272) -> (18.1341, 10.4718)
  line L3207 (47.5064, -0.5108) -> (37.29, -0.5108)
  line L3208 (43.6753, 0.5108) -> (43.6753, 0.2554)
  line L3209 (41.1212, 0.5108) -> (41.1212, 0.2554)
  line L3210 (47.5064, 1.2771) -> (37.29, 1.2771)
  line L3211 (46.2294, 0.5108) -> (46.2294, 0.2554)
  line L3212 (38.567, 0.5108) -> (38.567, 0.2554)
  line L3213 (37.29, 2.0434) -> (34.7358, 2.0434)
  line L3214 (36.0129, 3.0649) -> (36.0129, 2.8095)
  line L3215 (37.29, 3.8312) -> (34.7358, 3.8312)
  line L3216 (37.29, 4.5975) -> (34.7358, 4.5975)
  line L3217 (37.29, 6.3853) -> (34.7358, 6.3853)
  line L3218 (36.0129, 5.619) -> (36.0129, 5.3636)
  line L3219 (37.29, 7.1516) -> (34.7358, 7.1516)
  line L3220 (36.0129, 8.1731) -> (36.0129, 7.9177)
  line L3221 (37.29, 8.9394) -> (34.7358, 8.9394)
  line L3222 (37.29, 9.7057) -> (34.7358, 9.7057)
  line L3223 (37.29, 11.4935) -> (34.7358, 11.4935)
  line L3224 (36.0129, 10.7272) -> (36.0129, 10.4718)
  line L3225 (37.29, 12.2598) -> (34.7358, 12.2598)
  line L3226 (36.0129, 13.2813) -> (36.0129, 13.0259)
  line L3227 (37.29, 14.0476) -> (34.7358, 14.0476)
  line L3228 (37.29, 14.8139) -> (34.7358, 14.8139)
  line L3229 (19.4112, 12.2598) -> (16.8571, 12.2598)
  line L3230 (18.1341, 13.2813) -> (18.1341, 13.0259)
  line L3231 (19.4112, 14.0476) -> (16.8571, 14.0476)
  line L3232 (19.4112, 14.8139) -> (16.8571, 14.8139)
  line L3233 (19.4112, 16.6017) -> (16.8571, 16.6017)
  line L3234 (18.1341, 15.8354) -> (18.1341, 15.58)
  line L3235 (19.4112, 17.368) -> (16.8571, 17.368)
  line L3236 (19.4112, 19.1558) -> (16.8571, 19.1558)
  line L3237 (19.4112, 19.9221) -> (16.8571, 19.9221)
  line L3238 (18.1341, 18.3895) -> (18.1341, 18.1341)
  line L3239 (19.4112, 21.7099) -> (16.8571, 21.7099)
  line L3240 (18.1341, 20.9436) -> (18.1341, 20.6882)
  line L3241 (19.4112, 22.4762) -> (16.8571, 22.4762)
  line L3242 (18.1341, 23.4977) -> (18.1341, 23.2424)
  line L3243 (19.4112, 24.264) -> (16.8571, 24.264)
  line L3244 (19.4112, 25.0303) -> (16.8571, 25.0303)
  line L3245 (19.4112, 26.8181) -> (16.8571, 26.8181)
  line L3246 (18.1341, 26.0518) -> (18.1341, 25.7965)
  line L3247 (19.4112, 27.5844) -> (16.8571, 27.5844)
  line L3248 (19.4112, 29.3723) -> (16.8571, 29.3723)
  line L3249 (19.4112, 30.1386) -> (16.8571, 30.1386)
  line L3250 (18.1341, 28.606) -> (18.1341, 28.3506)
  line L3251 (24.9026, 21.3779) -> (22.3485, 21.3779)
  line L3252 (23.6255, 22.3996) -> (23.6255, 22.1441)
  line L3253 (24.9026, 23.1657) -> (22.3485, 23.1657)
  line L3254 (24.9026, 23.932) -> (22.3485, 23.932)
  line L3255 (24.9026, 25.7198) -> (22.3485, 25.7198)
  line L3256 (23.6255, 24.9537) -> (23.6255, 24.6982)
  line L3257 (24.9026, 10.855) -> (22.3485, 10.855)
  line L3258 (24.9026, 12.6428) -> (22.3485, 12.6428)
  line L3259 (24.9026, 13.4091) -> (22.3485, 13.4091)
  line L3260 (23.6255, 11.8766) -> (23.6255, 11.6213)
  line L3261 (24.9026, 15.1969) -> (22.3485, 15.1969)
  spline S1012 degree 3 poles (4.1377, 32.1817) (4.1377, 32.8447) (3.6002, 33.3822) (2.9373, 33.3822) knots 0 0 0 0 1 1 1 1
  line L3262 (4.1377, 32.1817) -> (4.1377, 32.8447) construction
  line L3263 (4.1377, 32.8447) -> (3.6002, 33.3822) construction
  line L3264 (3.6002, 33.3822) -> (2.9373, 33.3822) construction
  spline S1013 degree 3 poles (2.9373, 33.3822) (2.2743, 33.3822) (1.7368, 32.8447) (1.7368, 32.1817) knots 0 0 0 0 1 1 1 1
  line L3265 (2.9373, 33.3822) -> (2.2743, 33.3822) construction
  line L3266 (2.2743, 33.3822) -> (1.7368, 32.8447) construction
  line L3267 (1.7368, 32.8447) -> (1.7368, 32.1817) construction
  spline S1014 degree 3 poles (1.7368, 32.1817) (1.7368, 31.5188) (2.2743, 30.9813) (2.9373, 30.9813) knots 0 0 0 0 1 1 1 1
  line L3268 (1.7368, 32.1817) -> (1.7368, 31.5188) construction
  line L3269 (1.7368, 31.5188) -> (2.2743, 30.9813) construction
  line L3270 (2.2743, 30.9813) -> (2.9373, 30.9813) construction
  spline S1015 degree 3 poles (2.9373, 30.9813) (3.6002, 30.9813) (4.1377, 31.5188) (4.1377, 32.1817) knots 0 0 0 0 1 1 1 1
  line L3271 (2.9373, 30.9813) -> (3.6002, 30.9813) construction
  line L3272 (3.6002, 30.9813) -> (4.1377, 31.5188) construction
  line L3273 (4.1377, 31.5188) -> (4.1377, 32.1817) construction
  spline S1016 degree 3 poles (4.1377, 1.7878) (4.1377, 2.4507) (3.6002, 2.9882) (2.9373, 2.9882) knots 0 0 0 0 1 1 1 1
  line L3274 (4.1377, 1.7878) -> (4.1377, 2.4507) construction
  line L3275 (4.1377, 2.4507) -> (3.6002, 2.9882) construction
  line L3276 (3.6002, 2.9882) -> (2.9373, 2.9882) construction
  spline S1017 degree 3 poles (2.9373, 2.9882) (2.2743, 2.9882) (1.7368, 2.4507) (1.7368, 1.7878) knots 0 0 0 0 1 1 1 1
  line L3277 (2.9373, 2.9882) -> (2.2743, 2.9882) construction
  line L3278 (2.2743, 2.9882) -> (1.7368, 2.4507) construction
  line L3279 (1.7368, 2.4507) -> (1.7368, 1.7878) construction
  spline S1018 degree 3 poles (1.7368, 1.7878) (1.7368, 1.1249) (2.2743, 0.5874) (2.9373, 0.5874) knots 0 0 0 0 1 1 1 1
  line L3280 (1.7368, 1.7878) -> (1.7368, 1.1249) construction
  line L3281 (1.7368, 1.1249) -> (2.2743, 0.5874) construction
  line L3282 (2.2743, 0.5874) -> (2.9373, 0.5874) construction
  spline S1019 degree 3 poles (2.9373, 0.5874) (3.6002, 0.5874) (4.1377, 1.1249) (4.1377, 1.7878) knots 0 0 0 0 1 1 1 1
  line L3283 (2.9373, 0.5874) -> (3.6002, 0.5874) construction
  line L3284 (3.6002, 0.5874) -> (4.1377, 1.1249) construction
  line L3285 (4.1377, 1.1249) -> (4.1377, 1.7878) construction
  spline S1020 degree 3 poles (52.4103, 1.7878) (52.4103, 2.4507) (51.8729, 2.9882) (51.2099, 2.9882) knots 0 0 0 0 1 1 1 1
  line L3286 (52.4103, 1.7878) -> (52.4103, 2.4507) construction
  line L3287 (52.4103, 2.4507) -> (51.8729, 2.9882) construction
  line L3288 (51.8729, 2.9882) -> (51.2099, 2.9882) construction
  spline S1021 degree 3 poles (51.2099, 2.9882) (50.5469, 2.9882) (50.0095, 2.4507) (50.0095, 1.7878) knots 0 0 0 0 1 1 1 1
  line L3289 (51.2099, 2.9882) -> (50.5469, 2.9882) construction
  line L3290 (50.5469, 2.9882) -> (50.0095, 2.4507) construction
  line L3291 (50.0095, 2.4507) -> (50.0095, 1.7878) construction
  spline S1022 degree 3 poles (50.0095, 1.7878) (50.0095, 1.1249) (50.5469, 0.5874) (51.2099, 0.5874) knots 0 0 0 0 1 1 1 1
  line L3292 (50.0095, 1.7878) -> (50.0095, 1.1249) construction
  line L3293 (50.0095, 1.1249) -> (50.5469, 0.5874) construction
  line L3294 (50.5469, 0.5874) -> (51.2099, 0.5874) construction
  spline S1023 degree 3 poles (51.2099, 0.5874) (51.8729, 0.5874) (52.4103, 1.1249) (52.4103, 1.7878) knots 0 0 0 0 1 1 1 1
  line L3295 (51.2099, 0.5874) -> (51.8729, 0.5874) construction
  line L3296 (51.8729, 0.5874) -> (52.4103, 1.1249) construction
  line L3297 (52.4103, 1.1249) -> (52.4103, 1.7878) construction
  spline S1024 degree 3 poles (52.4103, 32.1817) (52.4103, 32.8447) (51.8729, 33.3822) (51.2099, 33.3822) knots 0 0 0 0 1 1 1 1
  line L3298 (52.4103, 32.1817) -> (52.4103, 32.8447) construction
  line L3299 (52.4103, 32.8447) -> (51.8729, 33.3822) construction
  line L3300 (51.8729, 33.3822) -> (51.2099, 33.3822) construction
  spline S1025 degree 3 poles (51.2099, 33.3822) (50.5469, 33.3822) (50.0095, 32.8447) (50.0095, 32.1817) knots 0 0 0 0 1 1 1 1
  line L3301 (51.2099, 33.3822) -> (50.5469, 33.3822) construction
  line L3302 (50.5469, 33.3822) -> (50.0095, 32.8447) construction
  line L3303 (50.0095, 32.8447) -> (50.0095, 32.1817) construction
  spline S1026 degree 3 poles (50.0095, 32.1817) (50.0095, 31.5188) (50.5469, 30.9813) (51.2099, 30.9813) knots 0 0 0 0 1 1 1 1
  line L3304 (50.0095, 32.1817) -> (50.0095, 31.5188) construction
  line L3305 (50.0095, 31.5188) -> (50.5469, 30.9813) construction
  line L3306 (50.5469, 30.9813) -> (51.2099, 30.9813) construction
  spline S1027 degree 3 poles (51.2099, 30.9813) (51.8729, 30.9813) (52.4103, 31.5188) (52.4103, 32.1817) knots 0 0 0 0 1 1 1 1
  line L3307 (51.2099, 30.9813) -> (51.8729, 30.9813) construction
  line L3308 (51.8729, 30.9813) -> (52.4103, 31.5188) construction
  line L3309 (52.4103, 31.5188) -> (52.4103, 32.1817) construction
  spline S1028 degree 3 poles (4.0865, 32.1817) (4.0865, 32.8164) (3.5719, 33.3312) (2.9373, 33.3312) knots 0 0 0 0 1 1 1 1
  line L3310 (4.0865, 32.1817) -> (4.0865, 32.8164) construction
  line L3311 (4.0865, 32.8164) -> (3.5719, 33.3312) construction
  line L3312 (3.5719, 33.3312) -> (2.9373, 33.3312) construction
  spline S1029 degree 3 poles (2.9373, 33.3312) (2.3026, 33.3312) (1.7878, 32.8164) (1.7878, 32.1817) knots 0 0 0 0 1 1 1 1
  line L3313 (2.9373, 33.3312) -> (2.3026, 33.3312) construction
  line L3314 (2.3026, 33.3312) -> (1.7878, 32.8164) construction
  line L3315 (1.7878, 32.8164) -> (1.7878, 32.1817) construction
  spline S1030 degree 3 poles (1.7878, 32.1817) (1.7878, 31.5471) (2.3026, 31.0325) (2.9373, 31.0325) knots 0 0 0 0 1 1 1 1
  line L3316 (1.7878, 32.1817) -> (1.7878, 31.5471) construction
  line L3317 (1.7878, 31.5471) -> (2.3026, 31.0325) construction
  line L3318 (2.3026, 31.0325) -> (2.9373, 31.0325) construction
  spline S1031 degree 3 poles (2.9373, 31.0325) (3.5719, 31.0325) (4.0865, 31.5471) (4.0865, 32.1817) knots 0 0 0 0 1 1 1 1
  line L3319 (2.9373, 31.0325) -> (3.5719, 31.0325) construction
  line L3320 (3.5719, 31.0325) -> (4.0865, 31.5471) construction
  line L3321 (4.0865, 31.5471) -> (4.0865, 32.1817) construction
  spline S1032 degree 3 poles (4.0865, 1.7878) (4.0865, 2.4225) (3.5719, 2.9373) (2.9373, 2.9373) knots 0 0 0 0 1 1 1 1
  line L3322 (4.0865, 1.7878) -> (4.0865, 2.4225) construction
  line L3323 (4.0865, 2.4225) -> (3.5719, 2.9373) construction
  line L3324 (3.5719, 2.9373) -> (2.9373, 2.9373) construction
  spline S1033 degree 3 poles (2.9373, 2.9373) (2.3026, 2.9373) (1.7878, 2.4225) (1.7878, 1.7878) knots 0 0 0 0 1 1 1 1
  line L3325 (2.9373, 2.9373) -> (2.3026, 2.9373) construction
  line L3326 (2.3026, 2.9373) -> (1.7878, 2.4225) construction
  line L3327 (1.7878, 2.4225) -> (1.7878, 1.7878) construction
  spline S1034 degree 3 poles (1.7878, 1.7878) (1.7878, 1.1532) (2.3026, 0.6385) (2.9373, 0.6385) knots 0 0 0 0 1 1 1 1
  line L3328 (1.7878, 1.7878) -> (1.7878, 1.1532) construction
  line L3329 (1.7878, 1.1532) -> (2.3026, 0.6385) construction
  line L3330 (2.3026, 0.6385) -> (2.9373, 0.6385) construction
  spline S1035 degree 3 poles (2.9373, 0.6385) (3.5719, 0.6385) (4.0865, 1.1532) (4.0865, 1.7878) knots 0 0 0 0 1 1 1 1
  line L3331 (2.9373, 0.6385) -> (3.5719, 0.6385) construction
  line L3332 (3.5719, 0.6385) -> (4.0865, 1.1532) construction
  line L3333 (4.0865, 1.1532) -> (4.0865, 1.7878) construction
  spline S1036 degree 3 poles (52.3592, 1.7878) (52.3592, 2.4225) (51.8445, 2.9373) (51.2099, 2.9373) knots 0 0 0 0 1 1 1 1
  line L3334 (52.3592, 1.7878) -> (52.3592, 2.4225) construction
  line L3335 (52.3592, 2.4225) -> (51.8445, 2.9373) construction
  line L3336 (51.8445, 2.9373) -> (51.2099, 2.9373) construction
  spline S1037 degree 3 poles (51.2099, 2.9373) (50.5753, 2.9373) (50.0605, 2.4225) (50.0605, 1.7878) knots 0 0 0 0 1 1 1 1
  line L3337 (51.2099, 2.9373) -> (50.5753, 2.9373) construction
  line L3338 (50.5753, 2.9373) -> (50.0605, 2.4225) construction
  line L3339 (50.0605, 2.4225) -> (50.0605, 1.7878) construction
  spline S1038 degree 3 poles (50.0605, 1.7878) (50.0605, 1.1532) (50.5753, 0.6385) (51.2099, 0.6385) knots 0 0 0 0 1 1 1 1
  line L3340 (50.0605, 1.7878) -> (50.0605, 1.1532) construction
  line L3341 (50.0605, 1.1532) -> (50.5753, 0.6385) construction
  line L3342 (50.5753, 0.6385) -> (51.2099, 0.6385) construction
  spline S1039 degree 3 poles (51.2099, 0.6385) (51.8445, 0.6385) (52.3592, 1.1532) (52.3592, 1.7878) knots 0 0 0 0 1 1 1 1
  line L3343 (51.2099, 0.6385) -> (51.8445, 0.6385) construction
  line L3344 (51.8445, 0.6385) -> (52.3592, 1.1532) construction
  line L3345 (52.3592, 1.1532) -> (52.3592, 1.7878) construction
  spline S1040 degree 3 poles (52.3592, 32.1817) (52.3592, 32.8164) (51.8445, 33.3312) (51.2099, 33.3312) knots 0 0 0 0 1 1 1 1
  line L3346 (52.3592, 32.1817) -> (52.3592, 32.8164) construction
  line L3347 (52.3592, 32.8164) -> (51.8445, 33.3312) construction
  line L3348 (51.8445, 33.3312) -> (51.2099, 33.3312) construction
  spline S1041 degree 3 poles (51.2099, 33.3312) (50.5753, 33.3312) (50.0605, 32.8164) (50.0605, 32.1817) knots 0 0 0 0 1 1 1 1
  line L3349 (51.2099, 33.3312) -> (50.5753, 33.3312) construction
  line L3350 (50.5753, 33.3312) -> (50.0605, 32.8164) construction
  line L3351 (50.0605, 32.8164) -> (50.0605, 32.1817) construction
  spline S1042 degree 3 poles (50.0605, 32.1817) (50.0605, 31.5471) (50.5753, 31.0325) (51.2099, 31.0325) knots 0 0 0 0 1 1 1 1
  line L3352 (50.0605, 32.1817) -> (50.0605, 31.5471) construction
  line L3353 (50.0605, 31.5471) -> (50.5753, 31.0325) construction
  line L3354 (50.5753, 31.0325) -> (51.2099, 31.0325) construction
  spline S1043 degree 3 poles (51.2099, 31.0325) (51.8445, 31.0325) (52.3592, 31.5471) (52.3592, 32.1817) knots 0 0 0 0 1 1 1 1
  line L3355 (51.2099, 31.0325) -> (51.8445, 31.0325) construction
  line L3356 (51.8445, 31.0325) -> (52.3592, 31.5471) construction
  line L3357 (52.3592, 31.5471) -> (52.3592, 32.1817) construction
  spline S1044 degree 3 poles (9.6418, 33.5866) (9.6418, 33.8334) (9.4415, 34.0334) (9.1948, 34.0334) knots 0 0 0 0 1 1 1 1
  line L3358 (9.6418, 33.5866) -> (9.6418, 33.8334) construction
  line L3359 (9.6418, 33.8334) -> (9.4415, 34.0334) construction
  line L3360 (9.4415, 34.0334) -> (9.1948, 34.0334) construction
  spline S1045 degree 3 poles (9.1948, 34.0334) (8.948, 34.0334) (8.7479, 33.8334) (8.7479, 33.5866) knots 0 0 0 0 1 1 1 1
  line L3361 (9.1948, 34.0334) -> (8.948, 34.0334) construction
  line L3362 (8.948, 34.0334) -> (8.7479, 33.8334) construction
  line L3363 (8.7479, 33.8334) -> (8.7479, 33.5866) construction
  spline S1046 degree 3 poles (8.7479, 33.5866) (8.7479, 33.3398) (8.948, 33.1395) (9.1948, 33.1395) knots 0 0 0 0 1 1 1 1
  line L3364 (8.7479, 33.5866) -> (8.7479, 33.3398) construction
  line L3365 (8.7479, 33.3398) -> (8.948, 33.1395) construction
  line L3366 (8.948, 33.1395) -> (9.1948, 33.1395) construction
  spline S1047 degree 3 poles (9.1948, 33.1395) (9.4415, 33.1395) (9.6418, 33.3398) (9.6418, 33.5866) knots 0 0 0 0 1 1 1 1
  line L3367 (9.1948, 33.1395) -> (9.4415, 33.1395) construction
  line L3368 (9.4415, 33.1395) -> (9.6418, 33.3398) construction
  line L3369 (9.6418, 33.3398) -> (9.6418, 33.5866) construction
  spline S1048 degree 3 poles (12.1959, 33.5866) (12.1959, 33.8334) (11.9957, 34.0334) (11.7489, 34.0334) knots 0 0 0 0 1 1 1 1
  line L3370 (12.1959, 33.5866) -> (12.1959, 33.8334) construction
  line L3371 (12.1959, 33.8334) -> (11.9957, 34.0334) construction
  line L3372 (11.9957, 34.0334) -> (11.7489, 34.0334) construction
  spline S1049 degree 3 poles (11.7489, 34.0334) (11.5021, 34.0334) (11.302, 33.8334) (11.302, 33.5866) knots 0 0 0 0 1 1 1 1
  line L3373 (11.7489, 34.0334) -> (11.5021, 34.0334) construction
  line L3374 (11.5021, 34.0334) -> (11.302, 33.8334) construction
  line L3375 (11.302, 33.8334) -> (11.302, 33.5866) construction
  spline S1050 degree 3 poles (11.302, 33.5866) (11.302, 33.3398) (11.5021, 33.1395) (11.7489, 33.1395) knots 0 0 0 0 1 1 1 1
  line L3376 (11.302, 33.5866) -> (11.302, 33.3398) construction
  line L3377 (11.302, 33.3398) -> (11.5021, 33.1395) construction
  line L3378 (11.5021, 33.1395) -> (11.7489, 33.1395) construction
  spline S1051 degree 3 poles (11.7489, 33.1395) (11.9957, 33.1395) (12.1959, 33.3398) (12.1959, 33.5866) knots 0 0 0 0 1 1 1 1